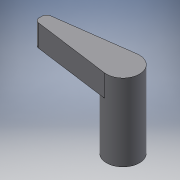
# Autodesk Inventor part: Pawl2
Saved by Autodesk Inventor 2019 (Build 230136000, 136)
## iProperties
Created: 2019-08-06
Part Number: Pawl2
Material: Generic
Document SubType Name: Modeling
Designer: aorfi
Density: 1 g/cm^3
Appearance: Default
Author: aorfi
Autodesk Inventor part; units mm, degrees
ref_plane "YZ Plane" through (0, 0, 0) normal (1, 0, 0) x (0, 1, 0)
ref_plane "XZ Plane" through (0, 0, 0) normal (0, 1, 0) x (-1, 0, 0)
ref_plane "XY Plane" through (0, 0, 0) normal (0, 0, 1) x (1, 0, 0)
sketch "Sketch1" plane through (0, 0, 0) normal (0, 1, 0) x (-1, 0, 0)
  circle A0 centre (0, 0) radius 1.5
  line L0 (0.2009, -1.4865) -> (7.5, -0.5)
  line L1 (7.5, 0.5) -> (0.2009, 1.4865)
  line L2 (7.5, 0.5) -> (7.5, -0.5)
  point P0 (7.5, 0)
  dimension "d2" = 3
  dimension "d13" = 7.5
  dimension "d14" = 1
  constraints: 6 end point, 2 point on circle, 2 tangent, 1 centre point, 1 coincident, 1 horizontal alignment, 1 midpoint, 1 vertical
  measures "d2" diameter of A0
  measures "d13" distance from line of A0.centre L2
  measures "d14" distance of L1.start L0.end
extrude "Extrusion1" add sketch "Sketch1" along normal mid plane 2
sketch "Sketch2" plane through (0, -1, 0) normal (0, 1, 0) x (1, 0, 0)
  arc A0 (-0.2009, -1.4865) -> (-0.2009, 1.4865) centre (0, 0) ccw projected
  circle A1 centre (0, 0) radius 1.5
  constraints: 1 centre point, 1 coincident, 1 concentric
extrude "Extrusion2" add sketch "Sketch2" against normal blind 5
fillet "Fillet1" radius 0.4 2 edges at (-7.5, 0, -0.5) (-7.5, 0, 0.5)
body "Solid1"
